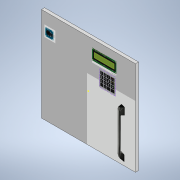
# Autodesk Inventor part: Part3
Saved by Autodesk Inventor 2022 (Build 260153000, 153)
## iProperties
Created: 2021-07-10
Part Number: Part3
Material: Generic
Document SubType Name: Modeling
Designer: Hp
Density: 1 g/cm^3
Appearance: Default
Author: Hp
Autodesk Inventor part; units mm, degrees
ref_plane "YZ Plane" through (0, 0, 0) normal (1, 0, 0) x (0, 1, 0)
ref_plane "XZ Plane" through (0, 0, 0) normal (0, 1, 0) x (-1, 0, 0)
ref_plane "XY Plane" through (0, 0, 0) normal (0, 0, 1) x (1, 0, 0)
sketch "Sketch1" plane through (0, 0, 0) normal (0, 0, 1) x (1, 0, 0)
  line L0 (-152.4, -152.4) -> (152.4, -152.4)
  line L1 (152.4, -152.4) -> (152.4, 152.4)
  line L2 (152.4, 152.4) -> (-152.4, 152.4)
  line L3 (-152.4, 152.4) -> (-152.4, -152.4)
  line L4 (-152.4, -152.4) -> (152.4, 152.4) construction
  line L5 (152.4, -152.4) -> (-152.4, 152.4) construction
  point P0 (0, 0)
  dimension "d0" = 304.8
  dimension "d1" = 304.8
  constraints: 12 end point, 2 midpoint, 2 parallel, 1 horizontal, 1 perpendicular
  measures "d0" distance of L2.end L1.end
  measures "d1" distance of L1.end L0.end
extrude "Extrusion1" add sketch "Sketch1" along normal blind 10
sketch "Sketch2" plane through (0, 0, 10) normal (0, 0, 1) x (1, 0, 0)
  point P0 (0, 0)
sketch "Sketch3" plane through (0, 0, 10) normal (0, 0, 1) x (1, 0, 0)
  line L0 (34.6646, 81.5942) -> (87.7523, 81.5942) construction
  line L1 (87.7523, 81.5942) -> (87.7523, 28.5065) construction
  line L2 (87.7523, 28.5065) -> (34.6646, 28.5065) construction
  line L3 (34.6646, 28.5065) -> (34.6646, 81.5942) construction
  point P0 (0, 0)
  constraints: 2 other
sketch "Sketch4" plane through (0, 0, 10) normal (0, 0, 1) x (1, 0, 0)
  line L0 (40.0273, 115.333) -> (77.7454, 115.333) construction
  line L1 (77.7454, 115.333) -> (77.7454, 86.7724) construction
  line L2 (77.7454, 86.7724) -> (40.0273, 86.7724) construction
  line L3 (40.0273, 86.7724) -> (40.0273, 115.333) construction
  point P0 (0, 0)
  constraints: 2 other
sketch "Sketch5" plane through (0, 0, 0) normal (0, 0, -1) x (-1, 0, 0)
  line L0 (-116.714, 59.7683) -> (-18.3595, 59.7683) construction
  line L1 (-18.3595, 59.7683) -> (-18.3595, 4.8054) construction
  line L2 (-18.3595, 4.8054) -> (-116.714, 4.8054) construction
  line L3 (-116.714, 4.8054) -> (-116.714, 59.7683) construction
  point P0 (0, 0)
  constraints: 2 other
sketch "Sketch6" plane through (0, 0, 0) normal (0, 0, -1) x (-1, 0, 0)
  point P0 (0, 0)
sketch "Sketch7" plane through (0, 0, 10) normal (0, 0, 1) x (1, 0, 0)
  point P0 (0, 0)
sketch "Sketch8" plane through (0, 0, 10) normal (0, 0, 1) x (1, 0, 0)
  line L0 (-142.6554, 115.4658) -> (-106.9983, 115.4658) construction
  line L1 (-106.9983, 115.4658) -> (-106.9983, 79.8087) construction
  line L2 (-106.9983, 79.8087) -> (-142.6554, 79.8087) construction
  line L3 (-142.6554, 79.8087) -> (-142.6554, 115.4658) construction
  point P0 (0, 0)
  constraints: 2 other
sketch "Sketch9" plane through (0, 0, 10) normal (0, 0, 1) x (1, 0, 0)
  line L0 (215.1591, 47.9318) -> (-4.6918, 47.9318) construction
  line L1 (-4.6918, 47.9318) -> (-4.6918, -171.9191) construction
  line L2 (-4.6918, -171.9191) -> (215.1591, -171.9191) construction
  line L3 (215.1591, -171.9191) -> (215.1591, 47.9318) construction
  point P0 (0, 0)
  constraints: 2 other
decal "Decal1"
decal "Decal2"
decal "Decal3"
decal "Decal4"
decal "Decal5"
decal "Decal6"
sketch "Sketch10" plane through (0, 0, 10) normal (0, 0, 1) x (1, 0, 0)
  point P0 (0, 0)
sketch "Sketch11" plane through (0, 0, 10) normal (0, 0, 1) x (1, 0, 0)
  point P0 (0, 0)
sketch "Sketch12" plane through (0, 0, 10) normal (0, 0, 1) x (1, 0, 0)
  point P0 (0, 0)
sketch "Sketch13" plane through (0, 0, 10) normal (0, 0, 1) x (1, 0, 0)
  line L0 (11.5465, 127.7808) -> (90.9215, 127.7808) construction
  line L1 (90.9215, 127.7808) -> (90.9215, 85.7121) construction
  line L2 (90.9215, 85.7121) -> (11.5465, 85.7121) construction
  line L3 (11.5465, 85.7121) -> (11.5465, 127.7808) construction
  point P0 (0, 0)
  constraints: 2 other
decal "Decal7"
decal "Decal8"
body "Solid1"
